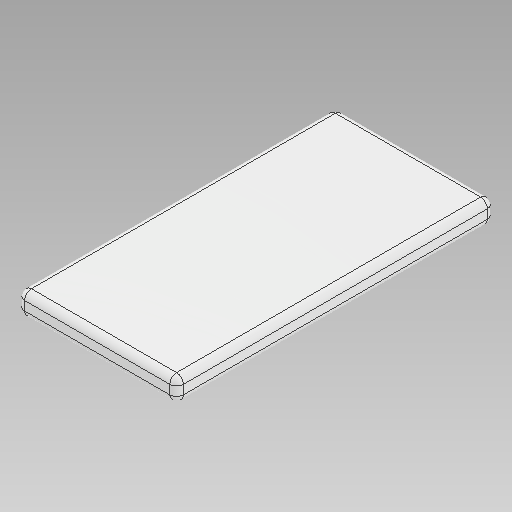
# Autodesk Inventor part: Powerbank
Saved by Autodesk Inventor 2020 (Build 240168000, 168)
## iProperties
Created: 2022-08-27
Part Number: Powerbank
Material: Acetal Resin, White
Document SubType Name: Modeling
Designer: Umair
Density: 1.425 g/cm^3
Appearance: Smooth - White
Author: Umair
Autodesk Inventor part; units mm, degrees
ref_plane "YZ Plane" through (0, 0, 0) normal (1, 0, 0) x (0, 1, 0)
ref_plane "XZ Plane" through (0, 0, 0) normal (0, 1, 0) x (-1, 0, 0)
ref_plane "XY Plane" through (0, 0, 0) normal (0, 0, 1) x (1, 0, 0)
sketch "Sketch1" plane through (0, 0, 0) normal (0, 1, 0) x (-1, 0, 0)
  line L0 (35, 70) -> (-35, 70)
  line L1 (-35, 70) -> (-35, -70)
  line L2 (-35, -70) -> (35, -70)
  line L3 (35, -70) -> (35, 70)
  line L4 (35, 70) -> (-35, -70) construction
  line L5 (-35, 70) -> (35, -70) construction
  point P0 (0, 0)
  dimension "d0" = 70
  dimension "d1" = 140
  constraints: 12 end point, 2 midpoint, 2 parallel, 1 horizontal, 1 perpendicular
  measures "d0" distance of L2.end L1.end
  measures "d1" distance of L1.end L0.end
extrude "Extrusion1" add sketch "Sketch1" along normal blind 10
fillet "Fillet1" radius 3 12 edges at (0, 10, -70) (0, 0, -70) (-35, 5, -70) (-35, 10, 0) (-35, 0, 0) (-35, 5, 70) (0, 10, 70) (0, 0, 70) (35, 5, 70) (35, 10, 0) (35, 5, -70) (35, 0, 0)
body "Solid1"
